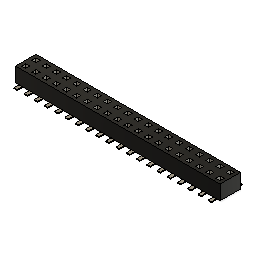
RPi SMT Connector (Autodesk Fusion 360 design; units mm, degrees)
Autodesk Fusion 360 part; units mm, degrees
sketch "Sketch1" plane through (0, 0, 0) normal (0, 1, 0) x (1, 0, 0)
  line L0 (1.27, -1.27) -> (-1.27, -1.27)
  line L1 (-1.27, -1.27) -> (-1.27, 1.27)
  line L2 (-1.27, 1.27) -> (1.27, 1.27)
  line L3 (1.27, 1.27) -> (1.27, -1.27)
  line L4 (1.27, -1.27) -> (-1.27, 1.27) construction
  line L5 (-1.27, -1.27) -> (1.27, 1.27) construction
  line L6 (0.5, -0.5) -> (-0.5, -0.5)
  line L7 (-0.5, -0.5) -> (-0.5, 0.5)
  line L8 (-0.5, 0.5) -> (0.5, 0.5)
  line L9 (0.5, 0.5) -> (0.5, -0.5)
  line L10 (0.5, -0.5) -> (-0.5, 0.5) construction
  line L11 (-0.5, -0.5) -> (0.5, 0.5) construction
  line L12 (1.27, 1.27) -> (-1.27, 1.27)
  line L13 (-1.27, 1.27) -> (-1.27, 3.81)
  line L14 (-1.27, 3.81) -> (1.27, 3.81)
  line L15 (1.27, 3.81) -> (1.27, 1.27)
  line L16 (1.27, 1.27) -> (-1.27, 3.81) construction
  line L17 (-1.27, 1.27) -> (1.27, 3.81) construction
  line L18 (0.5, 2.04) -> (-0.5, 2.04)
  line L19 (-0.5, 2.04) -> (-0.5, 3.04)
  line L20 (-0.5, 3.04) -> (0.5, 3.04)
  line L21 (0.5, 3.04) -> (0.5, 2.04)
  line L22 (0.5, 2.04) -> (-0.5, 3.04) construction
  line L23 (-0.5, 2.04) -> (0.5, 3.04) construction
  line L24 (-0.4, -0.93) -> (0.4, -0.93)
  line L25 (0.4, -0.93) -> (0.4, -2.53)
  line L26 (0.4, -2.53) -> (-0.4, -2.53)
  line L27 (-0.4, -2.53) -> (-0.4, -0.93)
  line L28 (0, -0.5) -> (0, -0.93) construction
  line L29 (-0.4, 5.07) -> (0.4, 5.07)
  line L30 (0.4, 5.07) -> (0.4, 3.47)
  line L31 (0.4, 3.47) -> (-0.4, 3.47)
  line L32 (-0.4, 3.47) -> (-0.4, 5.07)
  line L33 (0, 3.04) -> (0, 3.47) construction
  point P0 (0, 2.54)
  point P1 (0, 2.54)
  dimension "d1" = 2.54
  dimension "d2" = 2.54
  dimension "d3" = 1
  dimension "d4" = 1
  dimension "d5" = 2.54
  dimension "d6" = 2.54
  dimension "d7" = 1
  dimension "d8" = 1
  dimension "d9" = 1.6
  dimension "d10" = 0.8
  dimension "d11" = 1.6
  dimension "d12" = 0.8
  dimension "d13" = 7.6
  constraint horizontal L0
  constraint perpendicular L0 L1
  constraint parallel L0 L2
  constraint parallel L1 L3
  constraint coincident L4 origin
  constraint coincident L5 origin
  constraint horizontal L6
  constraint perpendicular L6 L7
  constraint parallel L6 L8
  constraint parallel L7 L9
  constraint coincident L10 origin
  constraint coincident L11 origin
  constraint horizontal L12
  constraint perpendicular L12 L13
  constraint parallel L12 L14
  constraint parallel L13 L15
  constraint coincident L16 P1
  constraint coincident L17 P1
  constraint collinear L2 L12
  constraint collinear L3 L15
  constraint horizontal L18
  constraint perpendicular L18 L19
  constraint parallel L18 L20
  constraint parallel L19 L21
  constraint coincident L22 P1
  constraint coincident L23 P1
  constraint coincident P1 P0
  constraint horizontal L24
  constraint vertical L25
  constraint horizontal L26
  constraint vertical L27
  constraint midpoint L6 L28.start
  constraint coincident L24 L28.end
  constraint perpendicular L24 L28
  constraint midpoint L24 L28.end
  constraint horizontal L29
  constraint vertical L30
  constraint horizontal L31
  constraint vertical L32
  constraint midpoint L20 L33.start
  constraint coincident L31 L33.end
  constraint perpendicular L31 L33
  constraint midpoint L31 L33.end
  constraint equal L28 L33
  measures "d1" distance of L1.end L2.end
  measures "d2" distance of L0.end L1.end
  measures "d3" distance of L7.end L8.end
  measures "d4" distance of L6.end L7.end
  measures "d5" distance of L13.end L14.end
  measures "d6" distance of L1.end L13.end
  measures "d7" distance of L19.end L20.end
  measures "d8" distance of L18.end L19.end
  measures "d9" distance of L24.start L26.end
  measures "d10" distance of L25.end L26.end
  measures "d11" distance of L29.start L31.end
  measures "d12" distance of L29.start L29.end
  measures "d13" distance of L26 L29
extrude "Extrude1" add sketch "Sketch1" along normal blind 0.2 contours L0 L25 L26 L27 | L0 L24 L25 L27 | L14 L30 L31 L32 | L14 L29 L30 L32 makes body 1 at (0.1333, 0, 1.9967) makes body 2 at (0.1333, 0, -4.0033)
extrude "Extrude2" add sketch "Sketch1" along normal blind 3.6 from surface at 0.2 contours L0 L1 L2 L3 L12 L24 L25 L27 | L0 L24 L25 L27 | L2 L12 L13 L14 L15 L30 L31 L32 | L14 L30 L31 L32 bodies 1 2
pattern_linear "R-Pattern1" count 20 spacing 2.54 along (1, 0, 0) of bodies 1 makes body 3 at (1.27, 1.4, -0.4233) makes body 4 at (4.0667, 3.8, -1.0133) makes body 5 at (6.6067, 3.8, -1.5267) makes body 6 at (9.1467, 3.8, -1.5267) makes body 7 at (11.6867, 3.8, -1.5267) makes body 8 at (16.2533, 3.8, -1.0133) makes body 9 at (16.7667, 3.8, -1.5267) makes body 10 at (19.3067, 3.8, -1.5267) makes body 11 at (21.8467, 3.8, -1.5267) makes body 12 at (24.3867, 3.8, -1.5267) makes body 13 at (26.9267, 3.8, -1.5267) makes body 14 at (29.4667, 3.8, -1.5267) makes body 15 at (34.0333, 3.8, -1.0133) makes body 16 at (34.5467, 3.8, -1.0133) makes body 17 at (37.0867, 3.8, -1.0133) makes body 18 at (39.6267, 3.8, -1.0133) makes body 19 at (42.1667, 3.8, -1.0133) makes body 20 at (44.7067, 3.8, -1.0133) makes body 21 at (49.53, 1.4, -2.1167)
combine "Combine1" operation add target body 5 tool bodies 1 7 12 17 3 13 4 19 6 9 14 18 21 20 11 8 16 15 10
equation "d11 = d9"
equation "d12 = d10"
